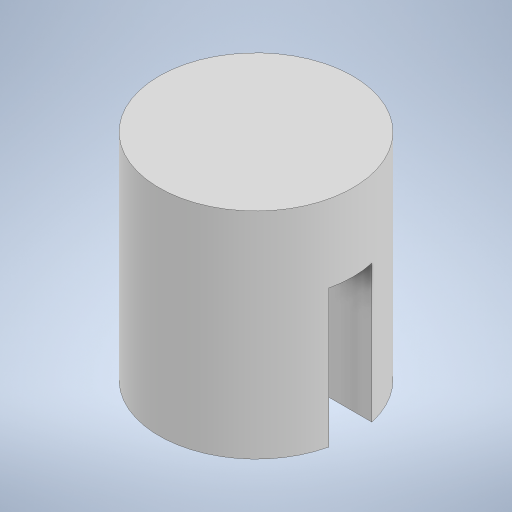
# Autodesk Inventor part: Piston Connector
Saved by Autodesk Inventor 2023 (Build 270158000, 158)
## iProperties
Created: 2023-02-24
Part Number: Piston Connector
Material: Generic
Document SubType Name: Modeling
Designer: tommy
Density: 1 g/cm^3
Appearance: Default
Author: tommy
Autodesk Inventor part; units mm, degrees
ref_plane "YZ Plane" through (0, 0, 0) normal (1, 0, 0) x (0, 1, 0)
ref_plane "XZ Plane" through (0, 0, 0) normal (0, 1, 0) x (-1, 0, 0)
ref_plane "XY Plane" through (0, 0, 0) normal (0, 0, 1) x (1, 0, 0)
sketch "Sketch1" plane through (0, 0, 0) normal (0, 1, 0) x (-1, 0, 0)
  circle A0 centre (0, 0) radius 1.7859
  circle A1 centre (0, 0) radius 2.3813
  line L0 (0, 0) -> (0, -0.3969)
  line L1 (0, -0.3969) -> (0, 0.3969)
  line L2 (0, 0.3969) -> (-2.3479, 0.3969)
  line L3 (-1.8581, 0.3969) -> (2.3479, 0.3969)
  line L4 (0, -0.3969) -> (2.3479, -0.3969)
  line L5 (1.8199, -0.3969) -> (-2.3479, -0.3969)
  point P0 (-1.7413, -0.3969)
  point P1 (1.7413, -0.3969)
  point P2 (1.7413, 0.3969)
  point P3 (-1.7413, 0.3969)
  dimension "d1" = 3.5719
  dimension "d2" = 4.7625
  dimension "d3" = 0.3969
  dimension "d4" = 0.7937
  constraints: 12 end point, 4 point on circle, 2 centre point, 2 point on line, 2 vertical, 1 coincident, 1 horizontal, 1 perpendicular
  measures "d1" diameter of A0
  measures "d2" diameter of A1
  measures "d3" distance of L0.start L0.end
  measures "d4" distance of L0.end L1.end
extrude "Extrusion1" add sketch "Sketch1" along normal blind 3.9624 contours A0 L4 L0 L1 L3 | L3 L2 A0 | A0 L5 L4 | L2 L1 L0 L5 A0
extrude "Extrusion2" cut sketch "Sketch1" along normal blind 2.54 contours A0 L4 L0 L1 L3 | L2 L1 L0 L5 A0
body "Solid1"
